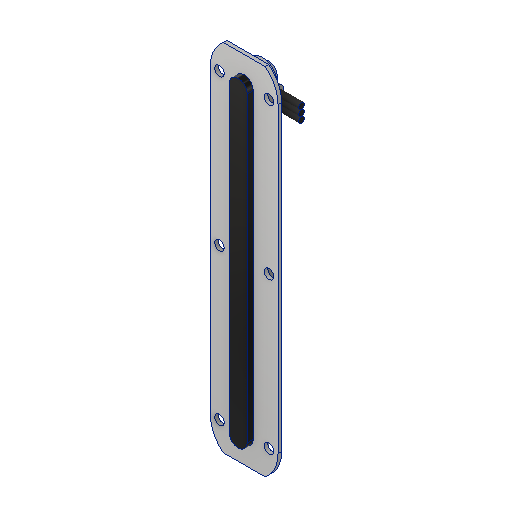
# Autodesk Inventor part: ASSEMBLY_Regolith_container_level_sensor
Saved by Autodesk Inventor 2025 (Build 290162010, 162A)
## iProperties
Created: 2018-09-16
Part Number: ASSEMBLY_Regolith_container_level_sensor
Material: Aluminum 6061
Document SubType Name: Modeling
Designer: Andrzej
Density: 2.7 g/cm^3
Appearance: Aluminum - Flat
Mass: 3.80456 g
Surface Area: 18.4484 cm^2
Volume: 1.40909 cm^3
Author: Andrzej
Autodesk Inventor part; units mm, degrees
ref_plane "YZ Plane" through (0, 0, 0) normal (1, 0, 0) x (0, 1, 0)
ref_plane "XZ Plane" through (0, 0, 0) normal (0, 1, 0) x (-1, 0, 0)
ref_plane "XY Plane" through (0, 0, 0) normal (0, 0, 1) x (1, 0, 0)
sketch "Sketch1" plane through (0, 0, 0) normal (0, 0, 1) x (1, 0, 0)
  line L0 (0, 54.4) -> (0, 4.4) construction
  line L1 (-1.5, 54.4) -> (-1.5, 4.4)
  line L2 (1.5, 4.4) -> (1.5, 54.4)
  arc A0 (1.5, 54.4) -> (-1.5, 54.4) centre (0, 54.4) ccw
  arc A1 (-1.5, 4.4) -> (1.5, 4.4) centre (0, 4.4) ccw
  line L3 (-5.6, 4.4) -> (-5.6, 54.4)
  line L4 (5.6, 54.4) -> (5.6, 4.4)
  line L5 (-4.1, 4.4) -> (-4.1, 54.4)
  arc A2 (4.1, 54.4) -> (-4.1, 54.4) centre (0, 54.4) ccw
  line L6 (4.1, 54.4) -> (4.1, 4.4)
  arc A3 (-4.1, 4.4) -> (4.1, 4.4) centre (0, 4.4) ccw
  line L7 (-2.5, 4.4) -> (-2.5, 54.4)
  arc A4 (2.5, 54.4) -> (-2.5, 54.4) centre (0, 54.4) ccw
  line L8 (2.5, 54.4) -> (2.5, 4.4)
  arc A5 (-2.5, 4.4) -> (2.5, 4.4) centre (0, 4.4) ccw
  arc A6 (5.6, 54.4) -> (3.4641, 58.8) centre (0, 54.4) ccw
  arc A7 (-3.4641, 58.8) -> (-5.6, 54.4) centre (0, 54.4) ccw
  arc A8 (-5.6, 4.4) -> (-3.4641, 0) centre (0, 4.4) ccw
  arc A9 (3.4641, 0) -> (5.6, 4.4) centre (0, 4.4) ccw
  line L9 (-3.4641, 0) -> (3.4641, 0)
  line L10 (-3.4641, 58.8) -> (3.4641, 58.8)
  point P0 (0, 0)
  point P1 (0, 1.5)
  point P2 (0, 29.4)
  point P3 (4.1, 29.4)
  point P4 (-4.1, 29.4)
  dimension "d0" = 3
  dimension "d1" = 50
  dimension "d2" = 4.1
  dimension "d3" = 2.6
  dimension "d4" = 1
  constraints: 24 end point, 21 point on circle, 10 centre point, 5 parallel, 4 coincident, 4 tangent, 3 midpoint, 1 horizontal, 1 vertical, 6 other
  measures "d0" diameter of A1
  measures "d1" distance of L0.start L0.end
  measures "d2" distance between parallel lines of L1 L3
  measures "d3" distance between parallel lines of L1 L5
  measures "d4" distance between parallel lines of L1 L7
extrude "Extrusion1" add sketch "Sketch1" along normal blind 1 contours A0 L2 A1 L1
extrude "Extrusion2" add sketch "Sketch1" against normal blind 4 contours A0 L2 A1 L1 | L7 A4 L8 A5
extrude "Extrusion3" add sketch "Sketch1" against normal blind 0.6 contours L3 A7 L10 A6 L4 A9 L9 A8 | L5 A2 L6 A3
chamfer "Chamfer1" distance 1 angle 45 4 edges at (2.5, 29.4, -4) (0, 1.9, -4) (-2.5, 29.4, -4) (0, 56.9, -4)
hole "Hole1" at (-4.1, 29.4, 0) at (4.1, 29.4, 0) at (-4.1, 54.4, 0) at (4.1, 54.4, 0) at (4.1, 4.4, 0) at (-4.1, 4.4, 0) direction (0, 0, -1) diameter 1.6 depth 8 tip angle 118
sketch "Sketch2" plane through (2.5, 4.4, -0.6) normal (1, 0, 0) x (0, 0, -1)
  line L0 (2.4, 50) -> (2.4, 0) projected
  line L1 (0, 50) -> (2.4, 50) projected
  line L2 (0, 50) -> (0, 0) projected
  line L3 (0, 0) -> (2.4, 0) projected
  line L4 (2.4, 48.8) -> (2.4, 46.8) construction
  line L5 (1.9, 48.8) -> (1.9, 46.8)
  line L6 (2.9, 46.8) -> (2.9, 48.8)
  arc A0 (2.9, 48.8) -> (1.9, 48.8) centre (2.4, 48.8) ccw
  arc A1 (1.9, 46.8) -> (2.9, 46.8) centre (2.4, 46.8) ccw
  line L7 (1.4, 48.8) -> (1.4, 46.8)
  arc A2 (1.4, 46.8) -> (3.4, 46.8) centre (2.4, 46.8) ccw
  line L8 (3.4, 46.8) -> (3.4, 48.8)
  arc A3 (3.4, 48.8) -> (1.4, 48.8) centre (2.4, 48.8) ccw
  circle A4 centre (2.4, 48.8) radius 0.5
  circle A5 centre (2.4, 46.8) radius 0.5
  circle A6 centre (2.4, 47.8) radius 0.5
  point P0 (-0.6, -4.4)
  dimension "d21" = 2
  dimension "d22" = 1
  dimension "d23" = 2.4
  dimension "d24" = 0
  dimension "d25" = 1.2
  dimension "d26" = 0.5
  dimension "d27" = 1
  dimension "d29" = 1
  constraints: 12 end point, 8 point on circle, 7 centre point, 4 tangent, 3 coincident, 2 parallel, 1 concentric, 1 midpoint, 1 vertical, 3 other
  measures "d21" distance of L4.start L4.end
  measures "d22" diameter of A1
  measures "d23" distance between parallel lines of L2 L0
  measures "d24" distance between parallel lines of L0 L4
  measures "d25" distance from line of L1 L4.start
  measures "d26" radial gap between concentric circles of A0 A3
  measures "d27" diameter of A4
  measures "d29" diameter of A6
extrude "Extrusion4" add sketch "Sketch2" against normal blind 1 contours A3 L8 A2 L0 A1 L6 A0 | L0 A0 L5 A1 A2 L7 A3
extrude "Extrusion5" add sketch "Sketch2" along normal mid plane 8 contours A0 A4 L0 | L0 A4 A0 | A6 L0 | L0 A6 | A5 A1 L0 | L0 A1 A5
body "Solid1"
